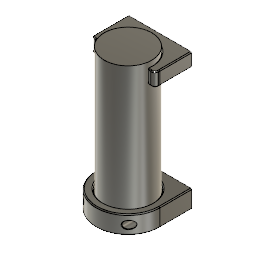
FireExtinguiserMount v7 (Autodesk Fusion 360 design; units mm, degrees)
Autodesk Fusion 360 part; units mm, degrees
note: some values were not read from the file. Set by a fixed rule: which sketch regions a step uses.
sketch "Sketch1" plane through (0, 0, 0) normal (0, 0, 1) x (1, 0, 0)
  circle A0 centre (0, 0) radius 33.147
  dimension "d1" = 66.294
  measures "d1" diameter of A0
extrude "Extrude1" add sketch "Sketch1" along normal blind 177.8 makes body 1
sketch "Sketch2" plane through (0, 0, 0) normal (0, 0, 1) x (1, 0, 0)
  circle A0 centre (0, 0) radius 34.29
  circle A1 centre (0, 0) radius 44.45
  line L0 (-44.45, 44.45) -> (44.45, 44.45)
  line L1 (44.45, 44.45) -> (44.45, 0)
  line L2 (44.45, 0) -> (-44.45, 0)
  line L3 (-44.45, 0) -> (-44.45, 44.45)
  dimension "d4" = 68.58
  dimension "d7" = 10.16
  measures "d4" diameter of A0
extrude "Extrude2" add sketch "Sketch2" against normal blind 19.05 separate body makes body 2
extrude "Extrude3" add sketch "Sketch2" along normal blind 6.35 contours A0 A1 L2 | A0 A1 L2 | A1 L0 L1 | A1 L0 L3 bodies 2
chamfer "Chamfer1" distance 1.27 angle 45 7 edges at (-31.9695, 12.3998, 6.35) (-44.45, 22.225, 6.35) (0, -44.45, 6.35) (44.45, 22.225, 6.35) (44.45, 22.225, -19.05) (0, -44.45, -19.05) (-44.45, 22.225, -19.05) on bodies 2
sketch "Sketch3" plane through (0, 44.45, 0) normal (0, 1, 0) x (-1, 0, 0)
  line L0 (43.18, -19.05) -> (44.45, -17.78)
  line L1 (44.45, -17.78) -> (44.45, 5.08)
  line L2 (44.45, 5.08) -> (43.18, 6.35)
  line L3 (43.18, 6.35) -> (-43.18, 6.35)
  line L4 (-43.18, 6.35) -> (-44.45, 5.08)
  line L5 (-44.45, 5.08) -> (-44.45, -17.78)
  line L6 (-44.45, -17.78) -> (-43.18, -19.05)
  line L7 (-43.18, -19.05) -> (43.18, -19.05)
  circle A0 centre (31.75, -6.35) radius 2.54
  circle A1 centre (-31.75, -6.35) radius 2.54
  circle A2 centre (-31.75, -6.35) radius 5.08
  circle A3 centre (31.75, -6.35) radius 5.08
  dimension "d13" = 5.08
  dimension "d14" = 5.08
  dimension "d15" = 12.7
  dimension "d16" = 12.7
  dimension "d17" = 10.16
  dimension "d18" = 10.16
  measures "d13" diameter of A0
  measures "d14" diameter of A1
  measures "d15" distance of L5
  measures "d16" distance of L1
  measures "d17" diameter of A2
  measures "d18" diameter of A3
extrude "Extrude4" cut sketch "Sketch3" against normal blind 134.62 from surface at -38.1 contours A0 | A1 | A2 | A3 bodies 2
extrude "Extrude5" cut sketch "Sketch3" against normal blind 38.1 contours A0 | A1 bodies 2
chamfer "Chamfer2" distance 2.54 angle 45 2 edges at (-29.3819, 6.35, -7.2685) (34.1181, 6.35, -7.2685) on bodies 2
chamfer "Chamfer3" distance 0.508 angle 45 2 edges at (-26.67, -35.56, -6.35) (36.83, -24.8868, -6.35) on bodies 2
ref_plane "WorkPlane1" through (0, 0, 152.4) normal (0, 0, 1) x (1, 0, 0)
sketch "Sketch4" plane through (0, 0, 152.4) normal (0, 0, 1) x (1, 0, 0)
  circle A0 centre (0, 0) radius 33.147
  circle A1 centre (0, 0) radius 44.45
  line L0 (-43.18, 44.45) -> (43.18, 44.45)
  line L1 (0, 44.45) -> (-44.45, 44.45)
  line L2 (-44.45, 44.45) -> (-44.45, 0)
  line L3 (44.45, 44.45) -> (44.45, 0)
  line L4 (43.18, 44.45) -> (44.45, 44.45)
  line L5 (0, 0) -> (-43.7747, -7.7187)
  line L6 (0, 0) -> (44.45, 0) construction
  line L7 (0, 0) -> (43.7747, -7.7187)
  line L8 (0, 0) -> (44.45, 0) construction
  dimension "d27" = 170
  dimension "d28" = 10
  measures "d27" angle of L5 L6
  measures "d28" angle of L7 L8
extrude "Extrude6" add sketch "Sketch4" along normal blind 19.05 separate body contours A0 A1 L5 L7 | A1 L0 L1 L2 | A1 L0 L3 L4 picked at (-40.46, 3.3636) makes body 3
fillet "Fillet1" radius 2.54 2 edges at (-32.6434, -5.7559, 161.925) (32.6434, -5.7559, 161.925) on bodies 3
fillet "Fillet2" radius 5.08 2 edges at (-43.7747, -7.7187, 161.925) (43.7747, -7.7187, 161.925) on bodies 3
sketch "Sketch5" plane through (0, 44.45, 0) normal (0, 1, 0) x (-1, 0, 0)
  line L0 (-44.45, 152.4) -> (44.45, 152.4)
  line L1 (44.45, 152.4) -> (44.45, 171.45)
  line L2 (44.45, 171.45) -> (-44.45, 171.45)
  line L3 (-44.45, 171.45) -> (-44.45, 152.4)
  circle A0 centre (-19.0047, 161.925) radius 2.54
  circle A1 centre (19.05, 161.925) radius 2.54
  line L4 (-44.4047, 152.4) -> (-44.4047, 171.45)
  circle A2 centre (-19.0047, 161.925) radius 5.08
  circle A3 centre (19.05, 161.925) radius 5.08
  dimension "d33" = 25.4
  dimension "d34" = 25.4
  dimension "d35" = 5.08
  dimension "d36" = 5.08
  dimension "d37" = 10.16
  dimension "d38" = 10.16
  dimension "d46" = 9.525
  measures "d35" diameter of A0
  measures "d36" diameter of A1
  measures "d37" diameter of A2
  measures "d38" diameter of A3
extrude "Extrude7" cut sketch "Sketch5" against normal blind 39.37 from surface at -12.7 contours A0 | A1 | A2 | A3 bodies 3
extrude "Extrude8" cut sketch "Sketch5" against normal blind 12.7 contours A0 | A1 bodies 3
chamfer "Chamfer4" distance 2.54 angle 45 2 edges at (-16.6819, 31.75, 161.0065) (21.3728, 31.75, 161.0065) on bodies 3
chamfer "Chamfer5" distance 1.27 angle 45 22 edges at (-44.45, 22.225, 171.45) (-44.4387, -1.0031, 171.45) (-42.5066, -5.7408, 171.45) (-36.7517, -6.4803, 171.45) (-33.4693, -5.2099, 171.45) (0, 33.147, 171.45) (33.4693, -5.2099, 171.45) (36.7517, -6.4803, 171.45) (42.5066, -5.7408, 171.45) (44.4387, -1.0031, 171.45) (44.45, 22.225, 171.45) (44.45, 22.225, 152.4) (44.4387, -1.0031, 152.4) (42.5066, -5.7408, 152.4) (36.7517, -6.4803, 152.4) (33.4693, -5.2099, 152.4) (0, 33.147, 152.4) (-33.4693, -5.2099, 152.4) (-36.7517, -6.4803, 152.4) (-42.5066, -5.7408, 152.4) (-44.4387, -1.0031, 152.4) (-44.45, 22.225, 152.4) on bodies 3
